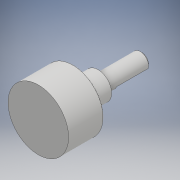
# Autodesk Inventor part: PotSensor
Saved by Autodesk Inventor 2018 (Build 220112000, 112)
## iProperties
Created: 2019-07-12
Part Number: PotSensor
Material: Generic
Document SubType Name: Modeling
Designer: aal_9
Density: 1 g/cm^3
Appearance: Default
Author: aal_9
Autodesk Inventor part; units mm, degrees
ref_plane "YZ Plane" through (0, 0, 0) normal (1, 0, 0) x (0, 1, 0)
ref_plane "XZ Plane" through (0, 0, 0) normal (0, 1, 0) x (-1, 0, 0)
ref_plane "XY Plane" through (0, 0, 0) normal (0, 0, 1) x (1, 0, 0)
sketch "Sketch1" plane through (0, 0, 0) normal (0, 1, 0) x (-1, 0, 0)
  circle A0 centre (0, 0) radius 11.1
  dimension "d0" = 22.2
  constraints: 1 centre point, 1 coincident
  measures "d0" diameter of A0
extrude "Extrusion1" add sketch "Sketch1" along normal blind 12.9
fillet "Fillet1" radius 0.3 1 edges at (11.1, 12.9, 0)
sketch "Sketch2" plane through (0, 12.9, 0) normal (0, 1, 0) x (1, 0, 0)
  circle A0 centre (0, 0) radius 5
  dimension "d4" = 10
  constraints: 1 centre point, 1 coincident
  measures "d4" diameter of A0
extrude "Extrusion2" add sketch "Sketch2" along normal blind 9
sketch "Sketch3" plane through (0, 21.9, 0) normal (0, 1, 0) x (1, 0, 0)
  circle A0 centre (0, 0) radius 3
  dimension "d9" = 6
  constraints: 1 centre point, 1 coincident
  measures "d9" diameter of A0
extrude "Extrusion3" add sketch "Sketch3" along normal blind 16
sketch "Sketch4" plane through (0, 12.9, 0) normal (0, 1, 0) x (1, 0, 0)
  circle A0 centre (-7.4, 0) radius 1.25
  circle A1 centre (0, 0) radius 3 projected
  circle A2 centre (0, 0) radius 5 projected
  dimension "d12" = 2.5
  dimension "d13" = 7.4
  dimension "d14" = 0
  constraints: 1 centre point
  measures "d12" diameter of A0
  measures "d13" distance of A0.centre A1.centre
  measures "d14" vertical distance of A2.centre A0.centre
extrude "Extrusion4" add sketch "Sketch4" along normal blind 1.2 contours A0
chamfer "Chamfer1" distance 0.5 angle 45 1 edges at (-3, 37.9, 0)
sketch "Sketch5" plane through (0, 37.9, 0) normal (0, 1, 0) x (1, 0, 0)
  line L0 (-3.6948, 5.5128) -> (4.164, 5.5128)
  line L1 (4.164, 5.5128) -> (4.164, 1)
  line L2 (4.164, 1) -> (-3.6948, 1)
  line L3 (-3.6948, 1) -> (-3.6948, 5.5128)
  circle A0 centre (0, 0) radius 3 projected
  dimension "d20" = 4
  constraints: 8 end point, 2 parallel, 1 horizontal, 1 perpendicular
extrude "Extrusion5" cut sketch "Sketch5" against normal blind 12 contours L0 L1 L2 A0 L3 | A0 L2 picked at (0.6732, 1.4061)
body "Solid1"
